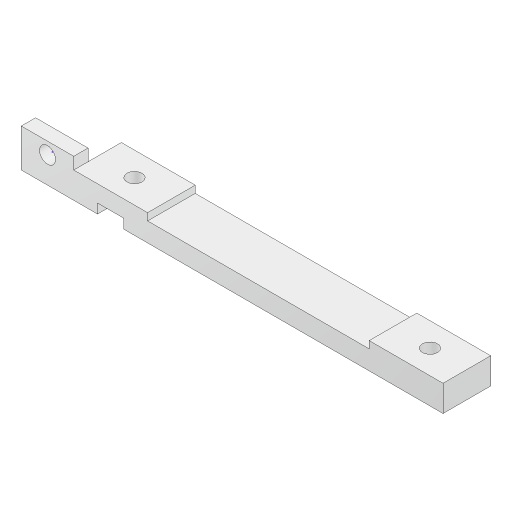
# Autodesk Inventor part: glue holder
Saved by Autodesk Inventor 2023 (Build 270158000, 158)
## iProperties
Created: 2023-10-31
Part Number: glue holder
Material: Aluminum 6061
Document SubType Name: Sheet Metal
Designer: PalumaCAD
Density: 2.7 g/cm^3
Sheet Metal Rule: Default_mm
Appearance: Aluminum - Flat
Mass: 9.7724 g
Surface Area: 27.502 cm^2
Volume: 3.61941 cm^3
Author: PalumaCAD
Autodesk Inventor part; units mm, degrees
ref_plane "YZ Plane" through (0, 0, 0) normal (1, 0, 0) x (0, 1, 0)
ref_plane "XZ Plane" through (0, 0, 0) normal (0, 1, 0) x (-1, 0, 0)
ref_plane "XY Plane" through (0, 0, 0) normal (0, 0, 1) x (1, 0, 0)
sketch "Sketch1" plane through (0, 0, 0) normal (0, 0, 1) x (1, 0, 0)
  line L0 (-5.5, -2.5) -> (5.5, -2.5)
  line L1 (5.5, -2.5) -> (5.5, 2.5)
  line L2 (5.5, 2.5) -> (-5.5, 2.5)
  line L3 (-5.5, 2.5) -> (-5.5, -2.5)
  line L4 (-5.5, -2.5) -> (5.5, 2.5) construction
  line L5 (5.5, -2.5) -> (-5.5, 2.5) construction
  circle A0 centre (0, 0) radius 1.25
  dimension "d0" = 11
  dimension "d1" = 5
  dimension "d2" = 2.5
  constraints: 12 end point, 2 midpoint, 2 parallel, 1 centre point, 1 coincident, 1 horizontal, 1 perpendicular
  measures "d0" distance of L2.end L1.end
  measures "d1" distance of L1.end L0.end
  measures "d2" diameter of A0
extrude "Extrusion1" add sketch "Sketch1" along normal blind 1
sketch "Sketch2" plane through (0, 0, 1) normal (0, 0, 1) x (1, 0, 0)
  line L0 (5.5, -2.5) -> (5.5, 2.5) projected
  line L1 (5.5, 0) -> (5.5, -2.5)
  line L2 (5.5, -2.5) -> (83, -2.5)
  line L3 (83, -2.5) -> (83, 0)
  line L4 (67.5, 0) -> (21, 0)
  line L5 (21, 0) -> (21, -1.5)
  line L6 (21, -1.5) -> (67.5, -1.5)
  line L7 (67.5, -1.5) -> (67.5, 0)
  line L8 (21, 0) -> (5.5, 0)
  line L9 (67.5, 0) -> (83, 0)
  point P0 (0, 0)
  dimension "d5" = 77.5
  dimension "d8" = 1.5
  dimension "d9" = 46.5
  constraints: 18 end point, 5 perpendicular, 2 parallel, 1 vertical
  measures "d5" distance of L2.end L0.start
  measures "d8" distance of L5.start L5.end
  measures "d9" distance of L6.end L5.end
extrude "Extrusion2" add sketch "Sketch2" against normal blind 10 contours L0 L8 L5 L6 L7 L9 L3 L2
sketch "Sketch3" plane through (-5.5, -2.5, 0) normal (0, -1, 0) x (1, 0, 0)
  line L0 (0, 0) -> (11, 0) projected
  line L1 (11, 0) -> (11, -9) projected
  line L2 (88.5, -9) -> (11, -9) projected
  line L3 (88.5, 1) -> (88.5, -9) projected
  line L4 (0, 1) -> (88.5, 1) projected
  line L5 (0, 0) -> (0, 1) projected
  point P0 (5.5, 0)
extrude "Extrusion3" add sketch "Sketch3" along normal blind 3
sketch "Sketch4" plane through (0, 0, 0) normal (0, 0, -1) x (-1, 0, 0)
  line L0 (-5.5, 2.5) -> (5.5, 2.5) projected
  line L1 (5.5, -5.5) -> (-5.5, -5.5) projected
  line L2 (5.5, 2.5) -> (-5.5, 2.5)
  line L3 (-5.5, 2.5) -> (-5.5, -5.5)
  line L4 (-5.5, -5.5) -> (5.5, -5.5)
  line L5 (5.5, -5.5) -> (5.5, 2.5)
  point P0 (0, 0)
  constraints: 8 end point, 2 parallel, 1 horizontal, 1 perpendicular
extrude "Extrusion4" add sketch "Sketch4" along normal blind 2
sketch "Sketch5" plane through (5.5, 0, 1) normal (0, 1, 0) x (1, 0, 0)
  point P0 (-5.5, 1)
sketch "Sketch6" plane through (0, 0, 0) normal (0, 0, 1) x (1, 0, 0)
  circle A0 centre (0, 0) radius 1.25
  dimension "d16" = 2.5
  constraints: 1 centre point, 1 coincident
  measures "d16" diameter of A0
hole "Hole1" at (0, 0, 0) direction (0, 0, -1) diameter 3.4 depth 4 tip angle 118 start extended yes clearance for "Hex Head Cap Screw ISO 24017" size "M3" standard "ISO"
sketch "Sketch7" plane through (5.5, 0, 1) normal (0, 1, 0) x (1, 0, 0)
  line L0 (0, 3) -> (0, 10) projected
  line L1 (15.5, 0) -> (15.5, 10) projected
  line L2 (0, 10) -> (15.5, 0)
  line L3 (0, 0) -> (0, 3) projected
  line L4 (15.5, 10) -> (0, 0)
  circle A0 centre (7.75, 5) radius 1.5
  point P0 (-5.5, 1)
  dimension "d24" = 3
  constraints: 4 end point, 1 centre point, 1 midpoint
  measures "d24" diameter of A0
hole "Hole2" at (13.25, 0, -4) direction (0, -1, 0) diameter 3.2 depth 10 tip angle 118 start extended yes clearance for "Hex Head Cap Screw ISO 24017" size "M3" standard "ISO"
sketch "Sketch8" plane through (67.5, 0, 1) normal (0, 1, 0) x (1, 0, 0)
  line L0 (-62, 10) -> (15.5, 10) projected
  line L1 (0.0027, 10) -> (15.5, -0.0212)
  line L2 (15.5, -0.0212) -> (15.5, 10)
  line L3 (0, 0) -> (0, 10) projected
  line L4 (15.5, 10) -> (0, 0)
  circle A0 centre (7.75, 5) radius 1.5
  point P0 (-67.5, 1)
  dimension "d32" = 3
  constraints: 6 end point, 1 centre point, 1 midpoint, 1 perpendicular, 1 point on line
  measures "d32" diameter of A0
hole "Hole3" at (75.25, 0, -4) direction (0, -1, 0) diameter 3.2 depth 10 tip angle 118 start extended yes clearance for "Hex Head Cap Screw ISO 24017" size "M3" standard "ISO"
sketch "Sketch9" plane through (0, 0, -9) normal (0, 0, -1) x (-1, 0, 0)
  line L0 (-83, -5.5) -> (5.5, -5.5) projected
  line L1 (-10.5, -5.5) -> (-16, -5.5)
  line L2 (-16, -5.5) -> (-16, -3.5)
  line L3 (-16, -3.5) -> (-10.5, -3.5)
  line L4 (-10.5, -3.5) -> (-10.5, -5.5)
  line L5 (-14.85, -5.5) -> (-14.85, 0) construction
  line L6 (-11.65, -5.5) -> (-11.65, 0) construction
  point P0 (0, 0)
  point P1 (-10.5, -4.5)
  point P2 (-16, -4.5)
  dimension "d40" = 5.5
  dimension "d41" = 3.2
  dimension "d42" = 1.15
  dimension "d43" = 2
  constraints: 8 end point, 2 midpoint, 2 parallel, 1 horizontal, 1 perpendicular, 1 point on line
  measures "d40" distance of point (-10.5, -4.5) point (-16, -4.5)
  measures "d41" distance between parallel lines of L6 L5
  measures "d42" distance from line of L5 point (-16, -4.5)
  measures "d43" distance between parallel lines of L0 L3
extrude "Extrusion5" cut sketch "Sketch9" against normal blind 10
equation "\"d42\" = -0.5 * d41 + 0.5 * d40"
equation "\"BendRadius\" = Thickness"
equation "\"BendReliefWidth\" = Thickness"
equation "\"BendReliefDepth\" = 0.5 * Thickness"
equation "\"CornerReliefSize\" = 4 * Thickness"
equation "\"MinimumRemnant\" = 2 * Thickness"
equation "\"TransitionRadius\" = BendRadius"
equation "\"JacobiRadiusSize\" = BendRadius"
equation "\"GapSize\" = Thickness"
equation "\"Thickness\" = 0.5"
body "Solid1"
